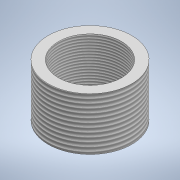
# Autodesk Inventor part: DS_lens_mount_adapter
Saved by Autodesk Inventor 2020 (Build 240168000, 168)
## iProperties
Created: 2019-07-08
Part Number: DS_lens_mount_adapter
Material: Generic
Document SubType Name: Modeling
Designer: Senior Design
Density: 1 g/cm^3
Appearance: Default
Author: Senior Design
Autodesk Inventor part; units mm, degrees
ref_plane "YZ Plane" through (0, 0, 0) normal (1, 0, 0) x (0, 1, 0)
ref_plane "XZ Plane" through (0, 0, 0) normal (0, 1, 0) x (-1, 0, 0)
ref_plane "XY Plane" through (0, 0, 0) normal (0, 0, 1) x (1, 0, 0)
sketch "Sketch1" plane through (0, 0, 0) normal (0, 1, 0) x (-1, 0, 0)
  circle A0 centre (0, 0) radius 7.94
  circle A1 centre (0, 0) radius 6
  dimension "d0" = 15.88
  dimension "d1" = 12
  constraints: 2 centre point, 2 coincident
  measures "d0" diameter of A0
  measures "d1" diameter of A1
extrude "Extrusion1" add sketch "Sketch1" along normal blind 10
thread "Thread2" size "5/8-32 UN" class "2A" standard "ANSI Unified Screw Threads" length 10
thread "Thread3" size "M12x0.5" class "6H" standard "ANSI Metric M Profile" length 10
body "Solid1"
